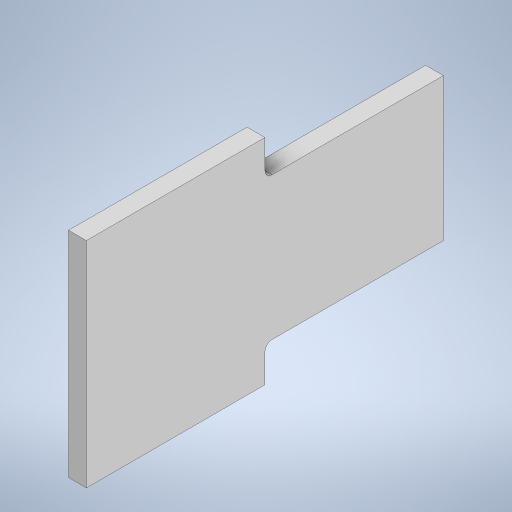
# Autodesk Inventor part: 05-23-2023 FEM
Saved by Autodesk Inventor 2023 (Build 270158000, 158)
## iProperties
Created: 2023-05-23
Part Number: 05-23-2023 FEM
Material: Generico
Document SubType Name: Modeling
Designer: Admin
Density: 1 g/cm^3
Appearance: Default
Author: Admin
Autodesk Inventor part; units mm, degrees
ref_plane "YZ Plane" through (0, 0, 0) normal (1, 0, 0) x (0, 1, 0)
ref_plane "XZ Plane" through (0, 0, 0) normal (0, 1, 0) x (-1, 0, 0)
ref_plane "XY Plane" through (0, 0, 0) normal (0, 0, 1) x (1, 0, 0)
sketch "Schizzo1" plane through (0, 0, 0) normal (0, 0, 1) x (1, 0, 0)
  line L0 (-5, 60) -> (5, 60)
  line L1 (5, 60) -> (5, -60)
  line L2 (5, -60) -> (-5, -60)
  line L3 (-5, -60) -> (-5, 60)
  line L4 (-5, 60) -> (5, -60) construction
  line L5 (5, 60) -> (-5, -60) construction
  line L6 (-5, 40) -> (5, 40)
  line L7 (5, 40) -> (5, -40)
  line L8 (5, -40) -> (-5, -40)
  line L9 (-5, -40) -> (-5, 40)
  line L10 (-5, 40) -> (5, -40) construction
  line L11 (5, 40) -> (-5, -40) construction
  line L12 (0, 0) -> (121.0573, 0)
  line L13 (0, 0) -> (0, 96.1234)
  dimension "d0" = 120
  dimension "d1" = 10
  dimension "d2" = 80
  constraints: 28 end point, 6 parallel, 4 midpoint, 3 horizontal, 2 perpendicular, 1 vertical
  measures "d0" distance of L2.end L0.start
  measures "d1" distance of L0.start L0.end
  measures "d2" distance between parallel lines of L8 L6
extrude "Estrusione1" add sketch "Schizzo1" along normal blind 100
extrude "Estrusione2" add sketch "Schizzo1" against normal blind 100 contours L6 L13 L12 L1 L8 L3 | L6 L1 L12 L13
fillet "Raccordo1" radius 4 2 edges at (0, 40, 0) (0, -40, 0)
